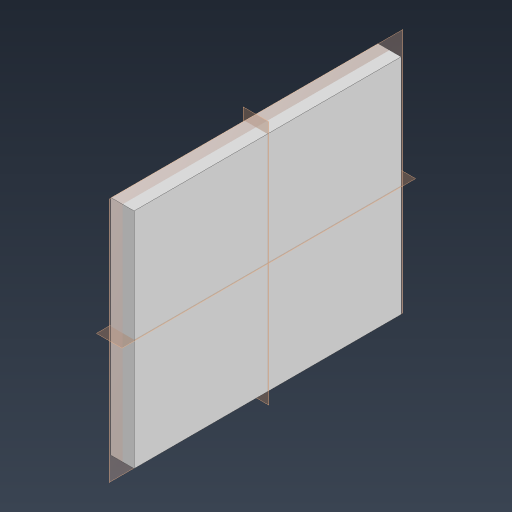
# Autodesk Inventor part: край задней стенки
Saved by Autodesk Inventor 2023.2 (Build 272271030, 271C)
## iProperties
Created: 2025-08-19
Part Number: край задней стенки
Material: Типовые
Document SubType Name: Modeling
Designer: Олег Коноваленко
Density: 1 g/cm^3
Appearance: По умолчанию
Author: Олег Коноваленко
Autodesk Inventor part; units mm, degrees
sketch "Эскиз1" plane through (0, 0, 0) normal (0, 1, 0) x (-1, 0, 0)
  line L0 (20, 230) -> (-20, 230)
  line L1 (-20, 230) -> (-20, -230)
  line L2 (-20, -230) -> (20, -230)
  line L3 (20, -230) -> (20, 230)
  line L4 (20, 230) -> (-20, -230) construction
  line L5 (-20, 230) -> (20, -230) construction
  point P0 (0, 0)
  dimension "d0" = 40
  dimension "d1" = 460
  constraints: 12 end point, 2 midpoint, 2 parallel, 1 horizontal, 1 perpendicular
  measures "d0" distance of L1.end L2.end
  measures "d1" distance of L0.end L1.end
extrude "Выдавливание1" add sketch "Эскиз1" along normal mid plane 384.5
